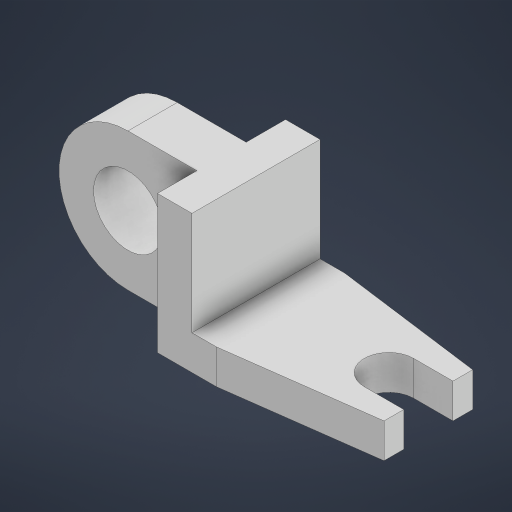
# Autodesk Inventor part: Część20
Saved by Autodesk Inventor 2023 (Build 270158000, 158)
## iProperties
Created: 2023-05-08
Part Number: Część20
Material: Ogólny
Document SubType Name: Modeling
Designer: Adam
Density: 1 g/cm^3
Appearance: Domyślna
Author: Adam
Autodesk Inventor part; units mm, degrees
ref_plane "YZ Plane" through (0, 0, 0) normal (1, 0, 0) x (0, 1, 0)
ref_plane "XZ Plane" through (0, 0, 0) normal (0, 1, 0) x (-1, 0, 0)
ref_plane "XY Plane" through (0, 0, 0) normal (0, 0, 1) x (1, 0, 0)
sketch "Szkic1" plane through (0, 0, 0) normal (0, 1, 0) x (-1, 0, 0)
  line L0 (0, 0) -> (-12, 0)
  line L1 (-12, 0) -> (-12, -26)
  line L2 (-12, -26) -> (0, -26)
  line L3 (0, -26) -> (0, 0)
  line L4 (-12, 0) -> (-42, -4)
  line L5 (-42, -4) -> (-42, -22)
  line L6 (-42, -22) -> (-12, -26)
  circle A0 centre (-34, -13) radius 5
  line L7 (-34, -18) -> (-42, -18)
  line L8 (-34, -8) -> (-42, -8)
  dimension "d0" = 12
  dimension "d1" = 26
  dimension "d2" = 18
  dimension "d3" = 30
  dimension "d4" = 10
  constraints: 18 end point, 3 perpendicular, 2 parallel, 2 point on circle, 2 point on line, 2 tangent, 1 centre point, 1 horizontal, 1 vertical
  measures "d0" distance of L2.end L1.end
  measures "d1" distance of L1.end L0.end
  measures "d2" distance of L4.end L5.end
  measures "d3" distance between parallel lines of L5 L1
  measures "d4" diameter of A0
extrude "Wyciągnięcie proste1" add sketch "Szkic1" along normal blind 7 contours L3 L2 L1 L0 | L1 L6 L5 L7 A0 L8 L4
sketch "Szkic2" plane through (0, 7, 0) normal (0, 1, 0) x (1, 0, 0)
  line L0 (0, 26) -> (0, 0) projected
  line L1 (0, 26) -> (7, 26)
  line L2 (7, 26) -> (7, 0)
  line L3 (7, 0) -> (0, 0)
  line L4 (0, 0) -> (0, 26)
  constraints: 8 end point, 2 parallel, 1 horizontal, 1 perpendicular
extrude "Wyciągnięcie proste2" add sketch "Szkic2" along normal blind 21
sketch "Szkic3" plane through (0, 0, -26) normal (-1, 0, 0) x (0, 0, 1)
  line L0 (8, 28) -> (18, 28)
  line L1 (18, 28) -> (18, 0)
  line L2 (18, 0) -> (8, 0)
  line L3 (8, 0) -> (8, 28)
  line L4 (0, 0) -> (0, 28) projected
  point P0 (26, 0)
  dimension "d9" = 10
  dimension "d10" = 8
  constraints: 8 end point, 2 parallel, 1 horizontal, 1 perpendicular
  measures "d9" distance of L1.end L2.end
  measures "d10" distance between parallel lines of L3 L4
extrude "Wyciągnięcie proste3" add sketch "Szkic3" along normal blind 28
sketch "Szkic4" plane through (0, 0, -8) normal (0, 0, 1) x (1, 0, 0)
  point P0 (0, 0)
  point P1 (-14, 14)
hole "Otwór1" at (-14, 14, -8) direction (0, 0, -1) diameter 14 end through all
full round fillet "Zaokrąglenie pełne1" first side at (-18.6667, 28, -14.6667) centre faces at (-28, 18.6667, -14.6667) second side at (17.6788, 0, -13.2009)
